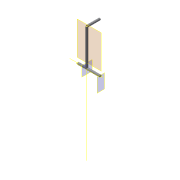
# Autodesk Inventor part: 00_Lightpath
Saved by Autodesk Inventor 2019 (Build 230136000, 136)
## iProperties
Created: 2019-10-10
Part Number: 00_Lightpath
Material: Generic
Document SubType Name: Modeling
Designer: diederichbenedict
Density: 1 g/cm^3
Appearance: Default
Author: diederichbenedict
Autodesk Inventor part; units mm, degrees
ref_plane "YZ Plane" through (0, 0, 0) normal (1, 0, 0) x (0, 1, 0)
ref_plane "XZ Plane" through (0, 0, 0) normal (0, 1, 0) x (-1, 0, 0)
ref_plane "Work Plane1" through (-0.2955, 151.1757, 22.2593) normal (-1, 0, 0) x (0, -1, 0)
sketch "Sketch1" plane through (-0.2955, 151.1757, 22.2593) normal (-1, 0, 0) x (0, -1, 0)
  arc A0 (59.8, 2) -> (63.9581, 11.1) centre (59.8, 7.5) ccw projected
  circle A1 centre (59.8, 7.5) radius 1.4305
  point P0 (151.1757, -22.2593)
  constraints: 1 centre point, 1 coincident
extrude "Extrusion1" add sketch "Sketch1" along normal blind 30
ref_plane "Work Plane2" through (-18.4955, 91.3757, 29.7593) normal (-1, 0, 0) x (0, -1, 0)
ref_plane "Work Plane4" through (-30.2955, 91.3757, 29.7593) normal (0, -1, 0) x (1, 0, 0)
ref_plane "Work Plane3" through (-0.2955, 73.8757, 22.2593) normal (0, -1, 0) x (1, 0, 0)
sketch "Sketch2" plane through (-30.2955, 91.3757, 29.7593) normal (0, -1, 0) x (1, 0, 0)
  line L0 (0, 1.4305) -> (0, -1.4305) projected
  line L1 (30, -1.4305) -> (30, 1.4305) projected
  circle A0 centre (11.8, 0) radius 1.4305
  line L2 (30, -1.4305) -> (0, -1.4305) projected
  line L3 (26.8, 6.34) -> (26.8, -6.34) projected
  point P0 (30.2955, -29.7593)
  dimension "d2" = 15
  constraints: 1 centre point, 1 tangent
  measures "d2" distance from line of L3 A0.centre
extrude "Extrusion2" add sketch "Sketch2" against normal blind 50
ref_plane "Work Plane6" through (-18.4955, 141.3757, 29.7593) normal (0, 0, 1) x (1, 0, 0)
ref_plane "Work Plane5" through (74.7045, 112.5257, 35.3593) normal (0, 0, 1) x (1, 0, 0)
sketch "Sketch3" plane through (-18.4955, 141.3757, 29.7593) normal (0, 0, 1) x (1, 0, 0)
  line L0 (1.4305, 0) -> (-1.4305, 0) projected
  circle A0 centre (0, 0) radius 1.4305
  line L1 (1.4305, -48.5695) -> (1.4305, 0) projected
  point P0 (18.4955, -141.3757)
  constraints: 1 centre point, 1 midpoint, 1 tangent
ref_plane "Work Plane7" through (-19.4482, 115.8757, 12.2593) normal (0, 0, 1) x (1, 0, 0)
extrude "Extrusion3" add sketch "Sketch3" against normal up to surface (17.5 mm away)
ref_plane "Work Plane10" through (-18.4955, 141.3757, 29.7593) normal (0, -0.7071, 0.7071) x (-1, 0, 0)
ref_plane "Work Plane9" through (-18.4955, 141.3757, 12.2593) normal (0, -1, 0) x (1, 0, 0)
ref_plane "Work Plane8" through (-57.7234, 76.1875, 20.0898) normal (0, -1, 0) x (1, 0, 0)
body "Solid1"
